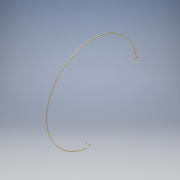
# Autodesk Inventor part: +XPanel_AntennaStowed-Y
Saved by Autodesk Inventor 2018 (Build 220112000, 112)
## iProperties
Created: 2018-07-10
Part Number: +XPanel_AntennaStowed-Y
Material: Titanium
Document SubType Name: Modeling
Designer: Bradley
Density: 4.51 g/cm^3
Appearance: Titanium
Author: Bradley
Autodesk Inventor part; units mm, degrees
ref_plane "XY Plane" through (0, 0, 0) normal (0, 0, 1) x (1, 0, 0)
sketch "Sketch1" plane through (0, 0, 0) normal (0, 1, 0) x (-1, 0, 0)
  circle A0 centre (0, 0) radius 0.2794
  dimension "d0" = 0.5588
  constraints: 1 centre point, 1 coincident
  measures "d0" diameter of A0
sketch "Sketch2" plane through (0, 0, 0) normal (0, 0, 1) x (1, 0, 0)
  line L0 (0, -3.5714) -> (0, 0)
  line L1 (-4.2178, 1) -> (-1.5, 1)
  circle A0 centre (-38.6, 2) radius 39 construction
  spline S0 degree 4 poles (-1.5, 1) (-1.2557, 1) (-0.7672, 1) (0, 0.8266) (0, 0.2755) (0, 0) knots 0 0 0 0 0 0.5 1 1 1 1 1
  dimension "d2" = 78
  dimension "d1" = 38.6
  dimension "d3" = 1
  dimension "d4" = 1.5
  dimension "d5" = 1
  dimension "d6" = 2.7178
  constraints: 4 end point, 2 horizontal, 2 vertical, 5 other
  measures "d1" distance from line of L0 point (-38.6, 2)
  measures "d3" distance from line of L0.end L1
  measures "d4" horizontal distance of L0.end L1.end
  measures "d5" distance from line of point (-38.6, 2) L1
  measures "d6" distance of L1.start L1.end
sweep "Sweep1" add profiles "Sketch1" path "Sketch2"
sketch "Sketch3" plane through (0, -3.5714, 0) normal (0, -1, 0) x (1, 0, 0)
  circle A0 centre (0, 0) radius 0.2794 projected
  point P0 (0, 0)
ref_plane "Work Plane1" through (-38.6, 2, 0) normal (0, 1, 0) x (-1, 0, 0)
sketch "Sketch5" plane through (-38.6, 2, 0) normal (0, 1, 0) x (-1, 0, 0)
  line L0 (-38.6, 38.6) -> (-41.3178, 38.6)
  point P0 (-38.6, 0)
  dimension "d18" = 38.6
  dimension "d19" = 2.7178
  constraints: 2 end point, 1 horizontal, 1 vertical alignment
  measures "d18" distance from line of point (-38.6, 0) L0
  measures "d19" distance of L0.start L0.end
coil "Coil2" sketch "Sketch3" operation add axis through (0, 2, 38.6) along (-1, 0, 0) pitch 1.25 turns 0.700941 hand right
sketch "Sketch6" plane through (-0.8762, 40.471, 45.0019) normal (0, 0.3033858, -0.9528678) x (-1, 0, 0)
  circle A0 centre (0, 0) radius 0.2794 projected
  point P0 (-0.8762, -52.2164)
  point P1 (-0.2794, 0)
  constraints: 1 horizontal alignment
ref_plane "Work Plane2" through (-0.8762, 40.471, 45.0019) normal (1, 0, 0) x (0, 1, 0)
sketch "Sketch7" plane through (-0.8762, 40.471, 45.0019) normal (1, 0, 0) x (0, 1, 0)
  circle A0 centre (-38.471, -6.4019) radius 39 construction
  circle A1 centre (-38.471, -6.4019) radius 39.3073 construction
  circle A2 centre (-38.471, -6.4019) radius 39.6147 construction
  arc A3 (-0.2302, -0.8184) -> (0, 0) centre (-0.9864, -0.1642) ccw
  arc A4 (-0.2302, -0.8184) -> (1.0637, -0.6295) centre (0.5261, -1.4727) ccw
  arc A5 (0.6146, 0.0508) -> (1.0637, -0.6295) centre (1.6013, 0.2137) ccw
  arc A6 (0.6146, 0.0508) -> (-0.2349, 3.9578) centre (-38.471, -6.4019) ccw
  point P0 (-40.471, -45.0019)
  dimension "d28" = 0.6147
  dimension "d29" = 0.3073
  dimension "d30" = 1
  dimension "d31" = 4
  constraints: 11 point on circle, 6 centre point, 4 equal radius, 1 coincident, 1 concentric, 1 tangent, 5 other
  measures "d28" radial gap between concentric circles of A0 A2
  measures "d30" radius of A3
sweep "Sweep2" add profiles "Sketch6" path "Sketch7"
equation "\"d18\" = d1"
equation "\"d19\" = d6"
equation "\"d28\" = 1.1 * d0"
equation "\"d29\" = 0.5 * d28"
body "Solid1"
